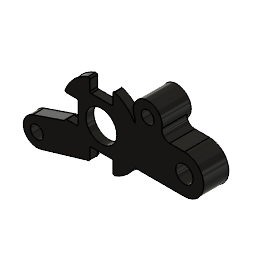
Dribbler Motor Holder End Par v1 (Autodesk Fusion 360 design; units mm, degrees)
part number: 2026-05-02-15-53-28-408
Autodesk Fusion 360 part; units mm, degrees
note: some values were not read from the file. Chosen so that the rebuilt part matches the saved one: which pieces of a blend or face edit are solid. Set by a fixed rule: which sketch regions a step uses.
sketch "Sketch1" plane through (0, 0, 0) normal (0, 0, 1) x (1, 0, 0)
  circle A0 centre (0, 0) radius 10
  circle A1 centre (0, 0) radius 4
  line L0 (0, 0) -> (-10, 0) construction
  line L1 (-10, 0) -> (-10, 3)
  line L2 (-10, 0) -> (-10, -3)
  line L3 (-10, 3) -> (-6, 3)
  line L4 (-6, 3) -> (-6, -3)
  line L5 (-6, -3) -> (-10, -3)
  line L6 (-10, -3) -> (-10, 3)
  line L7 (-3, -10) -> (-3, -6)
  line L8 (0, -10) -> (-3, -10)
  line L9 (3, -10) -> (-3, -10)
  line L10 (3, -6) -> (3, -10)
  line L11 (-3, -6) -> (3, -6)
  line L12 (10, -3) -> (6, -3)
  line L13 (10, 0) -> (10, -3)
  line L14 (10, 3) -> (10, -3)
  line L15 (6, 3) -> (10, 3)
  line L16 (6, -3) -> (6, 3)
  line L17 (3, 10) -> (3, 6)
  line L18 (0, 10) -> (3, 10)
  line L19 (-3, 10) -> (3, 10)
  line L20 (-3, 6) -> (-3, 10)
  line L21 (3, 6) -> (-3, 6)
  dimension "d1" = 20
  dimension "d2" = 8
  dimension "d3" = 3
  dimension "d4" = 3
  dimension "d5" = 4
  dimension "d6" = 6
  dimension "d8" = 360
  constraint coincident A0.centre A1.centre
  constraint coincident A0 L0.end
  constraint horizontal L0
  constraint perpendicular L0 L1
  constraint perpendicular L0 L2
  constraint horizontal L3
  constraint vertical L4
  constraint horizontal L5
  constraint vertical L6
  measures "d1" diameter of A0
  measures "d2" diameter of A1
  measures "d3" distance of L0.end L1.end
  measures "d4" distance of L0.end L2.end
  measures "d5" distance of L1.end L3.end
  measures "d6" distance of L1.end L2.end
extrude "Extrude1" add sketch "Sketch1" along normal blind 2 contours A0 L12 L15 L16 | A0 L3 L4 L5 L7 L10 L11 L12 L15 L16 L17 L20 L21
sketch "Sketch2" plane through (0, 0, 2) normal (0, 0, 1) x (1, 0, 0)
  circle A0 centre (0, 0) radius 4
  line L0 (3, 6) -> (-3, 6)
  line L1 (-3, 6) -> (-3, 9.5394)
  arc A1 (-3, 9.5394) -> (-9.5394, 3) centre (0, 0) ccw
  line L2 (-9.5394, 3) -> (-6, 3)
  line L3 (-6, 3) -> (-6, -3)
  line L4 (-6, -3) -> (-9.5394, -3)
  arc A2 (-9.5394, -3) -> (-3, -9.5394) centre (0, 0) ccw
  line L5 (-3, -9.5394) -> (-3, -6)
  line L6 (-3, -6) -> (3, -6)
  line L7 (3, -6) -> (3, -9.5394)
  arc A3 (3, -9.5394) -> (3, 9.5394) centre (0, 0) ccw
  line L8 (3, 9.5394) -> (3, 6)
  line L9 (0, 0) -> (21.5, 0)
  circle A4 centre (21.5, 0) radius 5
  line L10 (21.5, 0) -> (21.5, 5) construction
  line L11 (21.5, 5) -> (8.6603, 5)
  line L12 (21.5, -5) -> (8.6603, -5)
  circle A5 centre (21.5, 0) radius 2.25
  dimension "d11" = 21.5
  dimension "d12" = 10
  dimension "d13" = 4.5
  constraint coincident A0.centre A1.centre
  constraint horizontal L9
  constraint coincident L9.end A4.centre
  constraint coincident A4 L10.end
  constraint perpendicular L9 L10
  constraint coincident A3 L11.end
  constraint tangent A4 L11
  constraint coincident A4 L12.start
  constraint coincident A3 L12.end
  constraint tangent A4 L12
  constraint parallel L9 L12
  constraint concentric A4 A5
  measures "d11" distance of A0.centre L9.end
  measures "d12" diameter of A4
  measures "d13" diameter of A5
extrude "Extrude2" add sketch "Sketch2" against normal blind 6.5 contours A3 L9 A4 L11 | A3 L9 A4 L12 | A4
fillet "Fillet1" radius 0.35 12 edges at (3, 9.5394, 1) (-3, 9.5394, 1) (-9.5394, 3, 1) (-9.5394, -3, 1) (3, -9.5394, 1) (3, -6, 1) (3, 6, 1) (-3, 6, 1) (-6, 3, 1) (-6, -3, 1) (-3, -6, 1) (-3, -9.5394, 1)
sketch "Sketch3" plane through (0, 0, 2) normal (0, 0, 1) x (1, 0, 0)
  circle A0 centre (21.5, 0) radius 2.25
  circle A1 centre (0, 0) radius 4
  arc A2 (-3.4715, -9.3781) -> (-3, -9.0499) centre (-3.35, -9.0499) ccw
  line L0 (-3, -9.0499) -> (-3, -6.35)
  arc A3 (-2.65, -6) -> (-3, -6.35) centre (-2.65, -6.35) ccw
  line L1 (-2.65, -6) -> (2.65, -6)
  arc A4 (3, -6.35) -> (2.65, -6) centre (2.65, -6.35) ccw
  line L2 (3, -6.35) -> (3, -9.0499)
  arc A5 (3, -9.0499) -> (3.4715, -9.3781) centre (3.35, -9.0499) ccw
  arc A6 (3.4715, -9.3781) -> (8.6603, -5) centre (0, 0) ccw
  line L3 (8.6603, -5) -> (21.5, -5)
  arc A7 (21.5, -5) -> (21.5, 5) centre (21.5, 0) ccw
  line L4 (21.5, 5) -> (8.6603, 5)
  arc A8 (8.6603, 5) -> (3.4715, 9.3781) centre (0, 0) ccw
  arc A9 (3.4715, 9.3781) -> (3, 9.0499) centre (3.35, 9.0499) ccw
  line L5 (3, 9.0499) -> (3, 6.35)
  arc A10 (2.65, 6) -> (3, 6.35) centre (2.65, 6.35) ccw
  line L6 (2.65, 6) -> (-2.65, 6)
  arc A11 (-3, 6.35) -> (-2.65, 6) centre (-2.65, 6.35) ccw
  line L7 (-3, 6.35) -> (-3, 9.0499)
  arc A12 (-3, 9.0499) -> (-3.4715, 9.3781) centre (-3.35, 9.0499) ccw
  arc A13 (-3.4715, 9.3781) -> (-9.3781, 3.4715) centre (0, 0) ccw
  arc A14 (-9.3781, 3.4715) -> (-9.0499, 3) centre (-9.0499, 3.35) ccw
  line L8 (-9.0499, 3) -> (-6.35, 3)
  arc A15 (-6, 2.65) -> (-6.35, 3) centre (-6.35, 2.65) ccw
  line L9 (-6, 2.65) -> (-6, -2.65)
  arc A16 (-6.35, -3) -> (-6, -2.65) centre (-6.35, -2.65) ccw
  line L10 (-6.35, -3) -> (-9.0499, -3)
  arc A17 (-9.0499, -3) -> (-9.3781, -3.4715) centre (-9.0499, -3.35) ccw
  arc A18 (-9.3781, -3.4715) -> (-3.4715, -9.3781) centre (0, 0) ccw
  line L11 (0, 0) -> (0, -9.3371)
  line L12 (0, 0) -> (-16.7143, -9.65)
  line L13 (0, 0) -> (13.9, 0) construction
  circle A19 centre (-16.7143, -9.65) radius 1.65
  circle A20 centre (-16.7143, -9.65) radius 3.5
  line L14 (-16.7143, -9.65) -> (-18.4643, -6.6189)
  line L15 (-18.4643, -6.6189) -> (-9.8625, -1.6527)
  line L16 (-3.4715, -9.3781) -> (-15.7204, -13.0059)
  line L17 (-9.3781, -3.4715) -> (-17.8365, -6.3348)
  dimension "d18" = 150
  dimension "d19" = 19.3
  dimension "d20" = 3.3
  dimension "d21" = 7
  constraint coincident A1.centre A6.centre
  constraint parallel L0 L11
  constraint horizontal L13
  constraint coincident L12.end A19.centre
  constraint concentric A19 A20
  constraint coincident A20 L14.end
  constraint perpendicular L12 L14
  constraint coincident A18 L15.end
  constraint tangent A20 L15
  constraint coincident A2.start A18.end
  constraint coincident A20 L16.end
  constraint tangent A20 L16
  constraint coincident A17.end A18.start
  constraint coincident A20 L17.end
  constraint tangent A20 L17
  measures "d18" angle of L12 L13
  measures "d19" distance of A1.centre L12.end
  measures "d20" diameter of A19
  measures "d21" diameter of A20
extrude "Extrude3" add sketch "Sketch3" against normal blind 3 contours A18 L12 A20 L17 | A18 L12 A20 L16 | L12 A19 A20 L14 | L12 A19 A20 L14
fillet "Fillet2" radius 0.5 2 edges at (-3.4715, -9.3781, 1) (-9.3781, -3.4715, 1)
sketch "Sketch4" plane through (0, 0, 2) normal (0, 0, 1) x (1, 0, 0)
  circle A0 centre (-16.7143, -9.65) radius 1.65
  circle A1 centre (21.5, 0) radius 2.25
  circle A2 centre (0, 0) radius 4
  arc A3 (-3.3919, -9.3973) -> (-3, -9.0499) centre (-3.35, -9.0499) ccw
  line L0 (-3, -9.0499) -> (-3, -6.35)
  arc A4 (-2.65, -6) -> (-3, -6.35) centre (-2.65, -6.35) ccw
  line L1 (-2.65, -6) -> (2.65, -6)
  arc A5 (3, -6.35) -> (2.65, -6) centre (2.65, -6.35) ccw
  line L2 (3, -6.35) -> (3, -9.0499)
  arc A6 (3, -9.0499) -> (3.4715, -9.3781) centre (3.35, -9.0499) ccw
  arc A7 (3.4715, -9.3781) -> (8.6603, -5) centre (0, 0) ccw
  line L3 (8.6603, -5) -> (21.5, -5)
  arc A8 (21.5, -5) -> (21.5, 5) centre (21.5, 0) ccw
  line L4 (21.5, 5) -> (8.6603, 5)
  arc A9 (8.6603, 5) -> (3.4715, 9.3781) centre (0, 0) ccw
  arc A10 (3.4715, 9.3781) -> (3, 9.0499) centre (3.35, 9.0499) ccw
  line L5 (3, 9.0499) -> (3, 6.35)
  arc A11 (2.65, 6) -> (3, 6.35) centre (2.65, 6.35) ccw
  line L6 (2.65, 6) -> (-2.65, 6)
  arc A12 (-3, 6.35) -> (-2.65, 6) centre (-2.65, 6.35) ccw
  line L7 (-3, 6.35) -> (-3, 9.0499)
  arc A13 (-3, 9.0499) -> (-3.4715, 9.3781) centre (-3.35, 9.0499) ccw
  arc A14 (-3.4715, 9.3781) -> (-9.3781, 3.4715) centre (0, 0) ccw
  arc A15 (-9.3781, 3.4715) -> (-9.0499, 3) centre (-9.0499, 3.35) ccw
  line L8 (-9.0499, 3) -> (-6.35, 3)
  arc A16 (-6, 2.65) -> (-6.35, 3) centre (-6.35, 2.65) ccw
  line L9 (-6, 2.65) -> (-6, -2.65)
  arc A17 (-6.35, -3) -> (-6, -2.65) centre (-6.35, -2.65) ccw
  line L10 (-6.35, -3) -> (-9.0499, -3)
  arc A18 (-9.0499, -3) -> (-9.3854, -3.2505) centre (-9.0499, -3.35) ccw
  arc A19 (-9.7045, -3.582) -> (-9.3854, -3.2505) centre (-9.8648, -3.1084) ccw
  line L11 (-9.7045, -3.582) -> (-17.8365, -6.3348)
  arc A20 (-17.8365, -6.3348) -> (-15.7204, -13.0059) centre (-16.7143, -9.65) ccw
  line L12 (-15.7204, -13.0059) -> (-3.5938, -9.4143)
  arc A21 (-3.3919, -9.3973) -> (-3.5938, -9.4143) centre (-3.4518, -9.8937) ccw
  line L13 (0, 0) -> (12, 0)
  line L14 (12, 0) -> (12, 8)
  circle A22 centre (12, 8) radius 1.65
  circle A23 centre (12, 8) radius 3.75
  dimension "d28" = 12
  dimension "d29" = 8
  dimension "d30" = 3.3
  dimension "d37" = 7.5
  constraint coincident A2.centre A7.centre
  constraint horizontal L13
  constraint perpendicular L13 L14
  constraint coincident L14.end A22.centre
  constraint concentric A22 A23
  measures "d28" distance of A2.centre L13.end
  measures "d29" distance of L13.end L14.end
  measures "d30" diameter of A22
  measures "d37" diameter of A23
extrude "Extrude4" add sketch "Sketch4" against normal blind 7.5 contours L4 A23
fillet "Fillet5" radius 2 2 edges at (14.25, 5, -1.25) (9.75, 5, -1.25)
fillet "Fillet6" radius 1.25 2 edges at (8.6603, 5, -2.25) (8.6603, -5, -2.25)
fillet "Fillet7" radius 0.5 3 edges at (9.586, -4.4717, 0) (9.9757, 0.6973, 0) (8.7502, 4.9753, 0)
